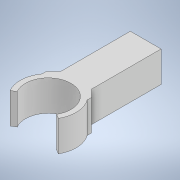
# Autodesk Inventor part: motor holder
Saved by Autodesk Inventor 2022 (Build 260153000, 153)
## iProperties
Created: 2021-11-11
Part Number: motor holder
Material: Generic
Document SubType Name: Modeling
Designer: a-dubs
Density: 1 g/cm^3
Appearance: Default
Author: a-dubs
Autodesk Inventor part; units mm, degrees
ref_plane "YZ Plane" through (0, 0, 0) normal (1, 0, 0) x (0, 1, 0)
ref_plane "XZ Plane" through (0, 0, 0) normal (0, 1, 0) x (-1, 0, 0)
ref_plane "XY Plane" through (0, 0, 0) normal (0, 0, 1) x (1, 0, 0)
sketch "Sketch1" plane through (0, 0, 0) normal (0, 1, 0) x (-1, 0, 0)
  line L0 (0, 0) -> (15, 0)
  line L1 (15, 0) -> (15, 34)
  line L2 (15, 34) -> (0, 34)
  line L3 (0, 34) -> (0, 0)
  line L4 (7.5, 34) -> (7.5, 36.5)
  line L5 (7.5, 36.5) -> (7.5, 47.61)
  circle A0 centre (7.5, 47.61) radius 11.11
  circle A1 centre (7.5, 47.61) radius 13.61
  line L6 (7.5, 47.61) -> (19.2866, 54.415)
  line L7 (7.5, 47.61) -> (21.11, 47.61) construction
  line L8 (7.5, 47.61) -> (-4.2866, 54.415)
  line L9 (7.5, 47.61) -> (21.11, 47.61) construction
  line L10 (15, 34) -> (18.5355, 37.5355)
  line L11 (15, 34) -> (20, 34) construction
  line L12 (18.5355, 37.5355) -> (18.5355, 39.6445)
  line L13 (0, 34) -> (-3.5355, 37.5355)
  line L14 (-3.5355, 37.5355) -> (-3.5355, 39.6445)
  point P0 (17.1215, 53.165)
  point P1 (-2.1215, 53.165)
  dimension "d0" = 15
  dimension "d1" = 34
  dimension "d2" = 2.5
  dimension "d3" = 11.11
  dimension "d4" = 30
  dimension "d5" = 150
  dimension "d6" = 5
  dimension "d7" = 45
  constraints: 30 end point, 4 horizontal, 4 point on circle, 3 equal length, 3 perpendicular, 3 vertical, 2 coincident, 2 symmetric about line, 1 centre point, 1 midpoint, 3 other
  measures "d0" distance of L0.start L0.end
  measures "d1" distance of L0.end L1.end
  measures "d2" distance of L4.start L4.end
  measures "d3" distance of L4.end L5.end
  measures "d4" angle of L7 L6
  measures "d5" angle of L9 L8
  measures "d6" distance of L1.end L10.end
  measures "d7" angle of L11 L10
extrude "Extrusion1" add sketch "Sketch1" along normal blind 15 contours L3 L2 L1 L0 | L13 L14 A1 L2 | L2 A1 L12 L10 | A1 L8 A0 L4 | L4 A0 L6 A1
equation "\"d8\" = d0"
body "Solid1"
